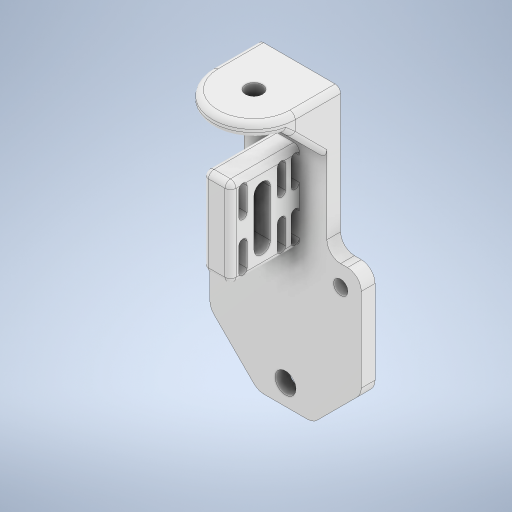
# Autodesk Inventor part: Gantry Plate
Saved by Autodesk Inventor 2023 (Build 270158000, 158)
## iProperties
Created: 2023-04-10
Part Number: Gantry Plate
Material: PC/ABS Plastic
Document SubType Name: Modeling
Designer: ethan
Density: 0.357273 g/cm^3
Appearance: Smooth - White
Author: ethan
Autodesk Inventor part; units mm, degrees
ref_plane "YZ Plane" through (0, 0, 0) normal (1, 0, 0) x (0, 1, 0)
ref_plane "XZ Plane" through (0, 0, 0) normal (0, 1, 0) x (-1, 0, 0)
ref_plane "XY Plane" through (0, 0, 0) normal (0, 0, 1) x (1, 0, 0)
sketch "Sketch1" plane through (0, 0, 0) normal (0, 1, 0) x (-1, 0, 0)
  line L0 (0, 0) -> (55, 0)
  line L1 (55, 0) -> (55, -55)
  line L2 (55, -55) -> (0, -55)
  line L3 (0, -55) -> (0, 0)
  line L4 (47.55, -7.45) -> (7.45, -7.45) construction
  line L5 (7.45, -7.45) -> (7.45, -47.55) construction
  line L6 (7.45, -47.55) -> (47.55, -47.55) construction
  line L7 (47.55, -47.55) -> (47.55, -7.45) construction
  circle A0 centre (47.55, -47.55) radius 2.6
  circle A1 centre (7.45, -47.55) radius 2.6
  circle A2 centre (27.5, -7.45) radius 3.8
  line L8 (0, -17.5) -> (17.5, 0)
  line L9 (37.5, 0) -> (55, -17.5)
  line L10 (12.5, -55) -> (42.5, -55)
  line L11 (42.5, -55) -> (42.5, -105.5)
  line L12 (42.5, -105.5) -> (12.5, -105.5)
  line L13 (12.5, -105.5) -> (12.5, -55)
  line L14 (0, -37.5) -> (55, -37.5) construction
  line L15 (0, -132.5) -> (55, -132.5) construction
  point P0 (42.5, -55)
  dimension "d0" = 55
  dimension "d1" = 55
  dimension "d2" = 40.1
  dimension "d3" = 40.1
  dimension "d6" = 5.2
  dimension "d7" = 5.2
  dimension "d8" = 7.45
  dimension "d9" = 7.45
  dimension "d14" = 7.6
  dimension "d55" = 20
  dimension "d56" = 10
  dimension "d81" = 30
  dimension "d90" = 12.5
  dimension "d113" = 10.05
  dimension "d114" = 68
  dimension "d115" = 95
  constraints: 32 end point, 7 point on line, 6 parallel, 6 perpendicular, 4 horizontal, 3 centre point, 2 coincident, 1 midpoint
  measures "d0" distance of L1.end L2.end
  measures "d1" distance of L0.end L1.end
  measures "d2" distance of L6.end L5.end
  measures "d3" distance of L5.end L4.end
  measures "d6" diameter of A0
  measures "d7" diameter of A1
  measures "d8" distance between parallel lines of L1 L7
  measures "d9" distance from line of L2 L5.end
  measures "d14" diameter of A2
  measures "d55" distance of L9.start L8.end
  measures "d56" horizontal distance of L8.end A2.centre
  measures "d81" distance of L11.end L12.end
  measures "d90" distance between parallel lines of L1 L11
  measures "d113" distance from line of L14 L5.end
  measures "d114" distance between parallel lines of L12 L14
  measures "d115" distance between parallel lines of L14 L15
extrude "Extrusion1" add sketch "Sketch1" along normal blind 5 contours L0 L9 L1 L2 L3 L8 | L2 L11 L12 L13
fillet "Fillet1" radius 5 8 edges at (-55, 2.5, -55) (0, 2.5, -55) (-55, 2.5, -17.5) (-37.5, 2.5, 0) (-17.5, 2.5, 0) (0, 2.5, -17.5) (-12.5, 2.5, -55) (-42.5, 2.5, -55)
sketch "Sketch12" plane through (0, 0, 0) normal (0, -1, 0) x (1, 0, 0)
  line L0 (-12.5, -105.5) -> (-42.5, -105.5) projected
  line L1 (-42.5, -105.5) -> (-42.5, -60) projected
  line L2 (-12.5, -105.5) -> (-42.5, -105.5)
  line L3 (-42.5, -105.5) -> (-42.5, -100.5)
  line L4 (-42.5, -100.5) -> (-12.5, -100.5)
  line L5 (-12.5, -100.5) -> (-12.5, -105.5)
  point P0 (0, 0)
  dimension "d83" = 5
  constraints: 8 end point, 2 parallel, 1 horizontal, 1 perpendicular, 1 point on line
  measures "d83" distance of L2.end L3.end
extrude "Extrusion15" add sketch "Sketch12" along normal blind 26.475
sketch "Sketch18" plane through (-12.5, 5, -105.5) normal (0, 0, -1) x (-1, 0, 0)
  line L0 (30, -5) -> (0, -5) construction
  line L1 (15, -5) -> (15, -16.475) construction
  circle A0 centre (15, -16.475) radius 3.1
  line L2 (30, -31.475) -> (30, 0) projected
  circle A1 centre (15, -16.475) radius 15 construction
  line L3 (0, -31.475) -> (0, 0) construction
  point P0 (-12.5, -5)
  point P1 (30, -18)
  dimension "d133" = 11.475
  dimension "d134" = 6.2
  constraints: 2 centre point, 2 coincident, 2 end point, 1 midpoint, 1 tangent, 1 vertical
  measures "d133" distance of L1.start L1.end
  measures "d134" diameter of A0
sketch "Sketch20" plane through (-55, 0, -19.5711) normal (-1, 0, 0) x (0, 0, 1)
  line L0 (-30.5789, 5) -> (-25.3789, 5) construction
  line L1 (-30.4289, 5) -> (0, 5) construction
  line L2 (-27.9789, 5) -> (-27.9789, 0) construction
  line L3 (-35.9789, -20.5) -> (-44.4789, -20.5) construction
  line L4 (-35.9789, -19) -> (-44.4789, -19)
  line L5 (-44.4789, -22) -> (-35.9789, -22)
  arc A0 (-35.9789, -22) -> (-35.9789, -19) centre (-35.9789, -20.5) ccw
  arc A1 (-44.4789, -19) -> (-44.4789, -22) centre (-44.4789, -20.5) ccw
  line L6 (-30.4289, 0) -> (0, 0) construction
  line L7 (-35.9789, -20.5) -> (-27.9789, -20.5) construction
  line L8 (-53.4789, -20.5) -> (-61.9789, -20.5) construction
  line L9 (-53.4789, -19) -> (-61.9789, -19)
  line L10 (-61.9789, -22) -> (-53.4789, -22)
  arc A2 (-53.4789, -22) -> (-53.4789, -19) centre (-53.4789, -20.5) ccw
  arc A3 (-61.9789, -19) -> (-61.9789, -22) centre (-61.9789, -20.5) ccw
  line L11 (-35.9789, -25.5) -> (-44.4789, -25.5) construction
  line L12 (-35.9789, -24) -> (-44.4789, -24)
  line L13 (-44.4789, -27) -> (-35.9789, -27)
  arc A4 (-35.9789, -27) -> (-35.9789, -24) centre (-35.9789, -25.5) ccw
  arc A5 (-44.4789, -24) -> (-44.4789, -27) centre (-44.4789, -25.5) ccw
  line L14 (-53.4789, -25.5) -> (-61.9789, -25.5) construction
  line L15 (-53.4789, -24) -> (-61.9789, -24)
  line L16 (-61.9789, -27) -> (-53.4789, -27)
  arc A6 (-53.4789, -27) -> (-53.4789, -24) centre (-53.4789, -25.5) ccw
  arc A7 (-61.9789, -24) -> (-61.9789, -27) centre (-61.9789, -25.5) ccw
  line L17 (-40.4289, 0) -> (-78.9289, 0) projected
  line L18 (-27.9789, 0) -> (-27.9789, -13.5) construction
  line L19 (-27.9789, -13.5) -> (-63.6214, -13.5) construction
  line L20 (-35.9789, -6.5) -> (-44.4789, -6.5) construction
  line L21 (-35.9789, -8) -> (-44.4789, -8)
  line L22 (-44.4789, -5) -> (-35.9789, -5)
  arc A8 (-35.9789, -8) -> (-35.9789, -5) centre (-35.9789, -6.5) ccw
  arc A9 (-44.4789, -5) -> (-44.4789, -8) centre (-44.4789, -6.5) ccw
  line L23 (-53.4789, -6.5) -> (-61.9789, -6.5) construction
  line L24 (-53.4789, -8) -> (-61.9789, -8)
  line L25 (-61.9789, -5) -> (-53.4789, -5)
  arc A10 (-53.4789, -8) -> (-53.4789, -5) centre (-53.4789, -6.5) ccw
  arc A11 (-61.9789, -5) -> (-61.9789, -8) centre (-61.9789, -6.5) ccw
  line L26 (-35.9789, -1.5) -> (-44.4789, -1.5) construction
  line L27 (-35.9789, -3) -> (-44.4789, -3)
  line L28 (-44.4789, 0) -> (-35.9789, 0)
  arc A12 (-35.9789, -3) -> (-35.9789, 0) centre (-35.9789, -1.5) ccw
  arc A13 (-44.4789, 0) -> (-44.4789, -3) centre (-44.4789, -1.5) ccw
  line L29 (-53.4789, -1.5) -> (-61.9789, -1.5) construction
  line L30 (-53.4789, -3) -> (-61.9789, -3)
  line L31 (-61.9789, 0) -> (-53.4789, 0)
  arc A14 (-53.4789, -3) -> (-53.4789, 0) centre (-53.4789, -1.5) ccw
  arc A15 (-61.9789, 0) -> (-61.9789, -3) centre (-61.9789, -1.5) ccw
  line L32 (-40.4789, -13.5) -> (-57.4789, -13.5) construction
  line L33 (-40.4789, -10.5) -> (-57.4789, -10.5)
  line L34 (-57.4789, -16.5) -> (-40.4789, -16.5)
  arc A16 (-40.4789, -16.5) -> (-40.4789, -10.5) centre (-40.4789, -13.5) ccw
  arc A17 (-57.4789, -10.5) -> (-57.4789, -16.5) centre (-57.4789, -13.5) ccw
  point P0 (19.5711, 0)
  point P1 (-40.2289, -20.5)
  point P2 (-57.7289, -20.5)
  point P3 (-40.2289, -25.5)
  point P4 (-57.7289, -25.5)
  point P5 (-40.2289, -6.5)
  point P6 (-57.7289, -6.5)
  point P7 (-40.2289, -1.5)
  point P8 (-57.7289, -1.5)
  point P9 (-48.9789, -13.5)
  point P10 (-60.4789, -13.5)
  point P11 (-37.4789, -13.5)
  point P12 (-34.4789, -20.5)
  point P13 (-63.4789, -20.5)
  point P14 (-15.2145, 5)
  dimension "d149" = 8.5
  dimension "d150" = 3
  dimension "d151" = 8
  dimension "d152" = 8.5
  dimension "d153" = 3
  dimension "d154" = 25.5
  dimension "d156" = 3
  dimension "d157" = 3
  dimension "d160" = 0
  dimension "d164" = 0
  dimension "d168" = 13.5
  dimension "d170" = 5.5
  dimension "d172" = 2
  dimension "d227" = 6
  dimension "d229" = 3
  dimension "d233" = 3
  constraints: 80 end point, 40 point on circle, 28 symmetric about line, 20 tangent, 18 centre point, 9 point on line, 8 parallel, 7 midpoint, 4 horizontal, 2 vertical, 1 collinear, 8 other
  measures "d149" distance of L3.start L3.end
  measures "d150" diameter of A1
  measures "d151" distance of L7.end L3.start
  measures "d152" distance of L8.start L8.end
  measures "d153" diameter of A3
  measures "d154" distance of L8.start L7.end
  measures "d156" diameter of A5
  measures "d157" diameter of A7
  measures "d160" horizontal distance of point (-57.729, -25.5) point (-57.729, -20.5)
  measures "d164" horizontal distance of point (-40.229, -25.5) point (-40.229, -20.5)
  measures "d168" distance of L2.end L18.end
  measures "d170" distance between parallel lines of L19 L4
  measures "d172" distance between parallel lines of L10 L15
  measures "d227" diameter of A17
  measures "d229" horizontal distance of point (-34.479, -20.5) point (-37.479, -13.5)
  measures "d233" horizontal distance of point (-63.479, -20.5) point (-60.479, -13.5)
sketch "Sketch21" plane through (0, 0, 0) normal (0, -1, 0) x (1, 0, 0)
  line L0 (-22.5, -52.65) -> (-32.5, -52.65)
  line L1 (-32.5, -52.65) -> (-32.5, -84.65)
  line L2 (-32.5, -84.65) -> (-22.5, -84.65)
  line L3 (-22.5, -84.65) -> (-22.5, -52.65)
  circle A0 centre (-7.45, -47.55) radius 2.6 projected
  line L4 (-42.5, -100.5) -> (-42.5, -60) projected
  line L5 (-12.5, -60) -> (-12.5, -100.5) projected
  line L6 (-42.5, -100.5) -> (-42.5, -90.5)
  line L7 (-12.5, -100.5) -> (-12.5, -90.5)
  line L8 (-12.5, -60) -> (-12.5, -105.5) projected
  point P0 (0, 0)
  dimension "d173" = 10
  dimension "d175" = 32
  dimension "d188" = 30
  dimension "d189" = 10
  dimension "d232" = 5.1
  constraints: 12 end point, 2 parallel, 2 point on line, 1 horizontal, 1 perpendicular
  measures "d173" distance of L1.end L2.end
  measures "d175" distance of L0.end L1.end
  measures "d188" distance between parallel lines of L4 L5
  measures "d189" distance between parallel lines of L4 L1
  measures "d232" distance from line of A0.centre L0
extrude "Extrusion22" add sketch "Sketch21" along normal blind 25 contours L3 L2 L1 L0
sketch "Sketch22" plane through (-32.5, 0, -84.65) normal (-1, 0, 0) x (0, 0, 1)
  line L0 (29.1, -19) -> (20.6, -19) projected
  arc A0 (20.6, -19) -> (20.6, -22) centre (20.6, -20.5) ccw projected
  line L1 (20.6, -22) -> (29.1, -22) projected
  arc A1 (29.1, -22) -> (29.1, -19) centre (29.1, -20.5) ccw projected
  arc A2 (20.6, -5) -> (20.6, -8) centre (20.6, -6.5) ccw projected
  line L2 (29.1, -8) -> (20.6, -8) projected
  line L3 (20.6, -5) -> (29.1, -5) projected
  arc A3 (29.1, -8) -> (29.1, -5) centre (29.1, -6.5) ccw projected
  line L4 (29.1, -3) -> (20.6, -3) projected
  arc A4 (20.6, 0) -> (20.6, -3) centre (20.6, -1.5) ccw projected
  line L5 (20.6, 0) -> (29.1, 0) projected
  arc A5 (29.1, -3) -> (29.1, 0) centre (29.1, -1.5) ccw projected
  arc A6 (3.1, 0) -> (3.1, -3) centre (3.1, -1.5) ccw projected
  line L6 (3.1, 0) -> (11.6, 0) projected
  arc A7 (11.6, -3) -> (11.6, 0) centre (11.6, -1.5) ccw projected
  line L7 (11.6, -3) -> (3.1, -3) projected
  line L8 (11.6, -8) -> (3.1, -8) projected
  arc A8 (3.1, -5) -> (3.1, -8) centre (3.1, -6.5) ccw projected
  line L9 (3.1, -5) -> (11.6, -5) projected
  arc A9 (11.6, -8) -> (11.6, -5) centre (11.6, -6.5) ccw projected
  line L10 (11.6, -19) -> (3.1, -19) projected
  arc A10 (11.6, -22) -> (11.6, -19) centre (11.6, -20.5) ccw projected
  line L11 (3.1, -22) -> (11.6, -22) projected
  arc A11 (3.1, -19) -> (3.1, -22) centre (3.1, -20.5) ccw projected
  line L12 (7.6, -16.5) -> (24.6, -16.5) projected
  arc A12 (24.6, -16.5) -> (24.6, -10.5) centre (24.6, -13.5) ccw projected
  line L13 (24.6, -10.5) -> (7.6, -10.5) projected
  arc A13 (7.6, -10.5) -> (7.6, -16.5) centre (7.6, -13.5) ccw projected
  point P0 (84.65, 0)
extrude "Extrusion23" cut sketch "Sketch22" against normal up to surface (10 mm away)
chamfer "Chamfer11" distance 15 angle 45 1 edges at (-27.5, 0, -100.5)
fillet "Fillet12" radius 15 2 edges at (-42.5, -26.475, -103) (-12.5, -26.475, -103)
fillet "Fillet13" radius 2 8 edges at (-32.5, -12.5, -84.65) (-22.5, -12.5, -84.65) (-32.5, -12.5, -52.65) (-22.5, -12.5, -52.65) (-32.5, -25, -68.65) (-22.5, -25, -68.65) (-27.5, -25, -52.65) (-27.5, -25, -84.65)
extrude "Extrusion27" cut sketch "Sketch18" against normal up to surface (5 mm away)
sketch "Sketch26" plane through (-27.5, -11.475, -100.5) normal (0, 0, 1) x (1, 0, 0)
  circle A0 centre (0, 0) radius 3.1 projected
  circle A1 centre (0, 0) radius 5.5
  point P0 (27.5, 11.475)
  dimension "d222" = 11
  constraints: 1 centre point, 1 coincident
  measures "d222" diameter of A1
extrude "Extrusion28" cut sketch "Sketch26" along normal blind 10 contours A0 | A1
fillet "Fillet15" radius 2 7 edges at (-36.7773, -23.2622, -100.5) (-42.3946, -13.2502, -98.7502) (-42.5, -5.7378, -91.2378) (-12.5, -5.7378, -91.2378) (-38.1067, -22.0817, -105.5) (-12.5, -3.2378, -105.5) (-42.5, -3.2378, -105.5)
equation "\"d1\" = d0"
equation "\"d3\" = d2"
equation "\"d8\" = -0.5 * d2 + 0.5 * d0"
equation "\"d9\" = -0.5 * d3 + 0.5 * d1"
equation "\"d90\" = -0.5 * d81 + 0.5 * d0"
body "Solid1"
